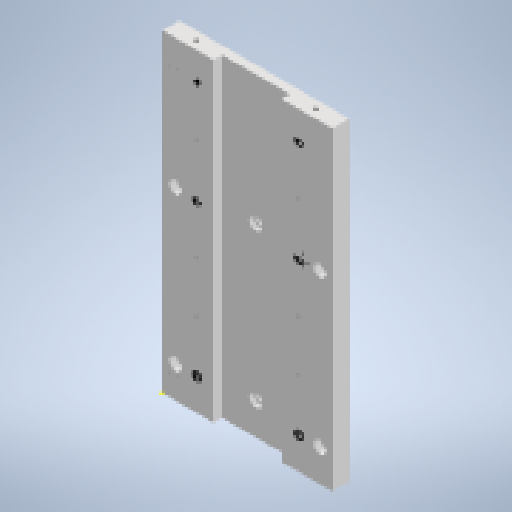
# Autodesk Inventor part: khung_doc
Saved by Autodesk Inventor 2023 (Build 270158000, 158)
## iProperties
Created: 2025-04-07
Part Number: khung_doc
Material: Generic
Document SubType Name: Modeling
Designer: huyqu
Density: 1 g/cm^3
Appearance: Default
Author: huyqu
Autodesk Inventor part; units mm, degrees
ref_plane "YZ Plane" through (0, 0, 0) normal (1, 0, 0) x (0, 1, 0)
ref_plane "XZ Plane" through (0, 0, 0) normal (0, 1, 0) x (-1, 0, 0)
ref_plane "XY Plane" through (0, 0, 0) normal (0, 0, 1) x (1, 0, 0)
sketch "Sketch1" plane through (0, 0, 0) normal (0, 0, 1) x (1, 0, 0)
  line L0 (0, 0) -> (200, 0)
  line L1 (200, 0) -> (200, 370)
  line L2 (200, 370) -> (0, 370)
  line L3 (0, 370) -> (0, 0)
  dimension "d0" = 200
  dimension "d1" = 370
  constraints: 8 end point, 2 parallel, 1 horizontal, 1 perpendicular
  measures "d0" distance of L1.end L2.end
  measures "d1" distance of L0.end L1.end
extrude "Extrusion1" add sketch "Sketch1" along normal blind 20
sketch "Sketch2" plane through (0, 0, 20) normal (0, 0, 1) x (1, 0, 0)
  line L0 (200, 370) -> (0, 370) projected
  line L1 (0, 0) -> (200, 0) projected
  line L2 (60, 370) -> (140, 370)
  line L3 (140, 370) -> (140, 0)
  line L4 (140, 0) -> (60, 0)
  line L5 (60, 0) -> (60, 370)
  line L6 (0, 370) -> (0, 0) projected
  dimension "d4" = 80
  dimension "d5" = 60
  constraints: 8 end point, 2 parallel, 2 point on line, 1 horizontal, 1 perpendicular
  measures "d4" distance between parallel lines of L3 L5
  measures "d5" distance between parallel lines of L5 L6
extrude "Extrusion2" cut sketch "Sketch2" against normal blind 10 contours L3 L1 L5 L0
sketch "Sketch4" plane through (0, 0, 20) normal (0, 0, 1) x (1, 0, 0)
  line L0 (-345, 211) -> (545, 211) projected
  line L1 (-345, 223.3) -> (545, 223.3) projected
  circle A0 centre (-305, 38) radius 4.5 projected
  line L2 (-345, 30) -> (545, 30) projected
  line L3 (-345, 43.3) -> (545, 43.3) projected
  line L4 (-18.5448, 211) -> (-18.5448, 223.3)
  line L5 (-12.5905, 30) -> (-12.5905, 43.3)
  line L6 (0, 370) -> (0, 0) projected
  line L7 (140, 0) -> (60, 0) projected
  line L8 (140, 370) -> (140, 0) projected
  line L9 (60, 370) -> (140, 370) projected
  line L10 (60, 0) -> (60, 370) projected
  line L11 (200, 0) -> (200, 370) projected
  line L12 (-345, 30.3) -> (545, 30.3) projected
  line L13 (-345, 238) -> (545, 238) projected
  line L14 (-345, 198) -> (545, 198) projected
  line L15 (-19.4055, 238) -> (-19.4055, 198)
  line L16 (-345, 18) -> (545, 18) projected
  line L17 (-345, 58) -> (545, 58) projected
  line L18 (-22.5041, 18) -> (-22.5041, 58)
  point P0 (15, 218)
  point P1 (100, 218)
  point P2 (185, 218)
  point P3 (15, 38)
  point P4 (100, 38)
  point P5 (185, 38)
  point P6 (100, 370)
  point P7 (-19.4055, 218)
  point P8 (-22.5041, 38)
  dimension "d15" = 15
  dimension "d17" = 15
  constraints: 8 end point, 8 point on line, 6 horizontal alignment, 4 vertical alignment, 3 midpoint, 3 vertical, 1 perpendicular
  measures "d15" distance from line of point (15, 218) L6
  measures "d17" distance from line of L11 point (185, 218)
hole "Hole2" at (15, 38, 20) at (185, 38, 20) at (185, 218, 20) at (15, 218, 20) direction (0, 0, -1) diameter 9 end through all counterbore diameter 15 counterbore depth 9
sketch "Sketch5" plane through (0, 0, 10) normal (0, 0, 1) x (1, 0, 0)
  circle A0 centre (15, 218) radius 4.5 projected
  circle A1 centre (185, 218) radius 4.5 projected
  circle A2 centre (15, 38) radius 4.5 projected
  circle A3 centre (185, 38) radius 4.5 projected
  line L0 (200, 370) -> (0, 370) projected
  line L1 (140, 0) -> (60, 0) projected
  line L2 (140, 370) -> (140, 0) projected
  line L3 (60, 370) -> (140, 370) projected
  line L4 (60, 0) -> (60, 370) projected
  point P0 (0, 0)
  point P1 (100, 218)
  point P2 (100, 38)
  point P3 (100, 370)
  point P4 (180.5, 218)
  point P5 (180.5, 218)
  point P6 (180.5, 38)
  point P7 (180.5, 38)
  point P8 (10.5, 218)
  point P9 (10.5, 218)
  point P10 (10.5, 38)
  point P11 (10.5, 38)
  constraints: 2 horizontal alignment, 2 vertical alignment, 1 midpoint
hole "Hole3" at (100, 38, 10) at (100, 218, 10) direction (0, 0, -1) diameter 9 end through all counterbore diameter 15 counterbore depth 5
sketch "Sketch6" plane through (0, 370, 0) normal (0, 1, 0) x (1, 0, 0)
  circle A0 centre (30, -10) radius 5.5 projected
  circle A1 centre (170, -10) radius 3.25 projected
  point P0 (0, 0)
hole "Hole4" at (30, 370, 10) at (170, 370, 10) direction (0, -1, 0) diameter 4.917 depth 15 tip angle 118 thread size "M6x1" class "6H" standard "ISO Metric profile"
sketch "Sketch7" plane through (0, 0, 0) normal (0, -1, 0) x (1, 0, 0)
  circle A0 centre (170, 10) radius 3.25 projected
  circle A1 centre (30, 10) radius 3.25 projected
  point P0 (0, 0)
hole "Hole5" at (30, 0, 10) at (170, 0, 10) direction (0, 1, 0) diameter 4.917 depth 17.1 tip angle 118 thread size "M6x1" class "6H" standard "ISO Metric profile"
sketch "Sketch9" plane through (0, 0, 20) normal (0, 0, 1) x (1, 0, 0)
  point P0 (0, 0)
sketch "Sketch10" plane through (0, 0, 20) normal (0, 0, 1) x (1, 0, 0)
  line L0 (0, 0) -> (200, 0) projected
  line L1 (18, 0) -> (18, 25)
  line L2 (0, 370) -> (0, 0) projected
  circle A0 centre (18, 25) radius 1
  line L3 (18, 25) -> (8.5, 25)
  circle A1 centre (8.5, 25) radius 1
  dimension "d48" = 18
  dimension "d49" = 2
  dimension "d50" = 9.5
  dimension "d51" = 25
  constraints: 4 end point, 2 centre point, 2 coincident, 1 horizontal, 1 point on line, 1 vertical
  measures "d48" distance between parallel lines of L1 L2
  measures "d49" diameter of A0
  measures "d50" distance of L3.start L3.end
  measures "d51" distance between parallel lines of L0 L3
hole "Hole6" at (8.5, 25, 20) at (18, 25, 20) direction (0, 0, -1) diameter 2.459 depth 9 thread size "M3x0.5" class "6H" standard "ISO Metric profile"
sketch "Sketch11" plane through (0, 0, 20) normal (0, 0, 1) x (1, 0, 0)
  line L0 (200, 370) -> (0, 370) projected
  line L1 (18, 370) -> (18, 338)
  line L2 (0, 370) -> (0, 0) projected
  circle A0 centre (18, 338) radius 1
  line L3 (18, 338) -> (8.5, 338)
  circle A1 centre (8.5, 338) radius 1
  point P0 (18, 354)
  dimension "d59" = 18
  dimension "d60" = 32
  dimension "d61" = 2
  dimension "d62" = 9.5
  constraints: 4 end point, 2 centre point, 2 coincident, 1 horizontal, 1 midpoint, 1 point on line, 1 vertical
  measures "d59" distance from line of point (18, 354) L2
  measures "d60" distance from line of L1.end L0
  measures "d61" diameter of A0
  measures "d62" distance of L3.start L3.end
hole "Hole7" at (8.5, 338, 20) at (18, 338, 20) direction (0, 0, -1) diameter 2.459 depth 9 thread size "M3x0.5" class "6H" standard "ISO Metric profile"
sketch "Sketch12" plane through (0, 0, 0) normal (0, 0, -1) x (-1, 0, 0)
  line L0 (-200, 370) -> (0, 370) projected
  line L1 (0, 370) -> (0, 0) projected
  line L2 (0, 0) -> (-200, 0) projected
  circle A0 centre (-100, 38) radius 4.5 projected
  circle A1 centre (-100, 218) radius 4.5 projected
  circle A2 centre (-185, 218) radius 4.5 projected
  circle A3 centre (-15, 38) radius 4.5 projected
  circle A4 centre (-185, 38) radius 4.5 projected
  circle A5 centre (-15, 218) radius 4.5 projected
  line L3 (-200, 0) -> (-200, 370) projected
  line L4 (0, 0) -> (-200, 0) projected
  line L5 (0, 370) -> (0, 0) projected
  line L6 (-200, 370) -> (0, 370) projected
  line L7 (-60, 370) -> (-140, 370) projected
  line L8 (0, 178) -> (-40, 178)
  line L9 (-40, 178) -> (-40, 143)
  line L10 (-40, 143) -> (0, 143)
  line L11 (0, 143) -> (0, 178)
  circle A6 centre (-21, 158) radius 7.5
  circle A7 centre (-15, 218) radius 4.5
  circle A8 centre (-185, 218) radius 4.5 projected
  point P0 (-179, 158)
  point P1 (0, 160.5)
  point P2 (-40, 160.5)
  point P3 (0, 160.5)
  dimension "d70" = 370
  dimension "d118" = 60
  dimension "d120" = 60
  constraints: 8 end point, 2 centre point
  measures "d70" distance of L2.end L0.start
  measures "d118" vertical distance of A6.centre A7.centre
  measures "d120" vertical distance of point (-179, 158) A8.centre
sketch "Sketch14" plane through (0, 0, 20) normal (0, 0, 1) x (1, 0, 0)
  point P0 (0, 0)
sketch "Sketch16" plane through (0, 0, 20) normal (0, 0, 1) x (1, 0, 0)
  arc A0 (40, 335) -> (40, 341) centre (40, 338) ccw
  arc A1 (155.25, 338) -> (164.75, 338) centre (160, 338) ccw
  arc A2 (155.25, 218) -> (164.75, 218) centre (160, 218) ccw
  arc A3 (35.25, 218) -> (44.75, 218) centre (40, 218) ccw
  circle A4 centre (40, 38) radius 4.75
  circle A5 centre (160, 38) radius 4.75
  point P0 (0, 0)
  constraints: 8 point on circle, 6 centre point, 20 other
sketch "Sketch17" plane through (0, 0, 20) normal (0, 0, 1) x (1, 0, 0)
  arc A0 (44.75, 278) -> (35.25, 278) centre (40, 278) ccw
  arc A1 (155.25, 278) -> (164.75, 278) centre (160, 278) ccw
  circle A2 centre (160, 158) radius 3
  circle A3 centre (160, 158) radius 4.75
  circle A4 centre (160, 98) radius 4.75
  circle A5 centre (40, 98) radius 4.75
  line L0 (60, 0) -> (60, 370) projected
  arc A6 (155.25, 338) -> (164.75, 338) centre (160, 338) ccw
  arc A7 (155.25, 218) -> (164.75, 218) centre (160, 218) ccw
  arc A8 (155.25, 278) -> (164.75, 278) centre (160, 278) ccw
  arc A9 (155.25, 158) -> (164.75, 158) centre (160, 158) ccw
  arc A10 (155.25, 218) -> (164.75, 218) centre (160, 218) ccw
  arc A11 (155.25, 98) -> (164.75, 98) centre (160, 98) ccw
  arc A12 (155.25, 158) -> (164.75, 158) centre (160, 158) ccw
  arc A13 (155.25, 38) -> (164.75, 38) centre (160, 38) ccw
  arc A14 (155.25, 98) -> (164.75, 98) centre (160, 98) ccw
  point P0 (0, 0)
  point P1 (40, 338)
  point P2 (40, 218)
  point P3 (40, 158)
  point P4 (40, 218)
  point P5 (40, 98)
  point P6 (40, 158)
  point P7 (40, 38)
  point P8 (40, 98)
  dimension "d15" = 15
  dimension "d17" = 15
  dimension "d97" = 60
  dimension "d100" = 60
  dimension "d105" = 60
  dimension "d108" = 60
  constraints: 22 point on circle, 15 centre point, 11 coincident, 4 vertical, 70 other
  measures "d97" distance of point (40, 278) point (40, 338)
  measures "d100" distance of point (40, 278) point (40, 218)
  measures "d105" distance of A1.start A6.start
  measures "d108" distance of A1.start A7.start
hole "Hole10" at (40, 278, 20) at (160, 278, 20) at (40, 338, 20) at (40, 218, 20) at (40, 158, 20) at (40, 98, 20) at (40, 38, 20) at (160, 338, 20) at (160, 218, 20) at (160, 158, 20) at (160, 98, 20) at (160, 38, 20) direction (0, 0, -1) diameter 4.134 depth 13 thread size "M5x0.8" class "6H" standard "ISO Metric profile"
sketch "Sketch18" plane through (0, 0, 0) normal (-1, 0, 0) x (0, 0, 1)
  line L0 (0, 153.5413) -> (0, 162.4587) projected
  line L1 (0, 158) -> (20, 158)
  line L2 (20, 160.067) -> (20, 155.933) projected
  line L3 (10, 162.4587) -> (10, 153.5413) projected
  line L4 (10, 158) -> (10, 152.5)
  circle A0 centre (10, 152.5) radius 1.5
  line L5 (10, 158) -> (10, 163.5)
  circle A1 centre (10, 163.5) radius 1.5
  point P0 (0, 0)
  point P1 (10, 158)
  dimension "d121" = 5.5
  dimension "d122" = 3
  dimension "d123" = 5.5
  dimension "d124" = 3
  constraints: 6 end point, 4 midpoint, 2 centre point, 2 coincident, 1 collinear, 1 point on line
  measures "d121" distance of L4.start L4.end
  measures "d122" diameter of A0
  measures "d123" distance of point (10, 158) L5.end
  measures "d124" diameter of A1
hole "Hole11" at (0, 163.5, 10) at (0, 152.5, 10) direction (1, 0, 0) diameter 2.459 depth 12 tip angle 118 thread size "M3x0.5" class "6H" standard "ISO Metric profile"
body "Solid1"
